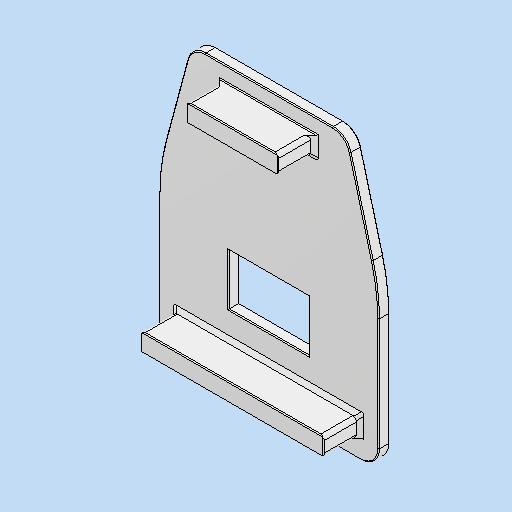
# Autodesk Inventor part: tc-back-panel
Saved by Autodesk Inventor 2025 (Build 290162000, 162)
## iProperties
Created: 2025-06-05
Part Number: tc-back-panel
Material: ABS Plastic
Document SubType Name: Modeling
Designer: queezz
Density: 1.06 g/cm^3
Appearance: Smooth - White
Author: queezz
Autodesk Inventor part; units mm, degrees
ref_plane "YZ Plane" through (0, 0, 0) normal (1, 0, 0) x (0, 1, 0)
ref_plane "XZ Plane" through (0, 0, 0) normal (0, 1, 0) x (-1, 0, 0)
ref_plane "XY Plane" through (0, 0, 0) normal (0, 0, 1) x (1, 0, 0)
sketch "Sketch1" plane through (0, 0, 0) normal (0, 0, 1) x (1, 0, 0)
  line L0 (-60, 75) -> (60, 75)
  line L1 (60, 75) -> (60, -75)
  line L2 (60, -75) -> (-60, -75)
  line L3 (-60, -75) -> (-60, 75)
  point P0 (0, 0)
  point P1 (60, 0)
  point P2 (0, 75)
  dimension "d0" = 120
  dimension "d1" = 150
  constraints: 8 end point, 2 midpoint, 2 parallel, 1 horizontal, 1 horizontal alignment, 1 perpendicular, 1 vertical alignment
  measures "d0" distance of L0.start L0.end
  measures "d1" distance of L0.end L1.end
extrude "Extrusion1" add sketch "Sketch1" along normal blind 6
sketch "Sketch2" plane through (0, 0, 6) normal (0, 0, 1) x (1, 0, 0)
  line L0 (-22, -11.7654) -> (22, -11.7654)
  line L1 (22, -11.7654) -> (22, -39.7654)
  line L2 (22, -39.7654) -> (-22, -39.7654)
  line L3 (-22, -39.7654) -> (-22, -11.7654)
  point P0 (0, 0)
  point P1 (0, -11.7654)
  dimension "d4" = 44
  dimension "d5" = 28
  constraints: 8 end point, 2 parallel, 1 horizontal, 1 midpoint, 1 perpendicular, 1 vertical alignment
  measures "d4" distance of L0.start L0.end
  measures "d5" distance of L0.end L1.end
extrude "PowerPlug" cut sketch "Sketch2" against normal through all
sketch "Sketch3" plane through (0, 0, 6) normal (0, 0, 1) x (1, 0, 0)
  line L0 (22, -11.7654) -> (22, -39.7654) projected
  line L1 (22, -39.7654) -> (-22, -39.7654) projected
  line L2 (-22, -39.7654) -> (-22, -11.7654) projected
  line L3 (-22, -11.7654) -> (22, -11.7654) projected
  line L4 (-60, -75) -> (60, -75) projected
  line L5 (60, -75) -> (60, 75) projected
  line L6 (60, 75) -> (-60, 75) projected
  line L7 (-60, 75) -> (-60, -75) projected
  line L8 (-60, 9.6891) -> (-42.5, 75)
  line L9 (42.5, 75) -> (60, 9.6891)
  line L10 (-42.5, 75) -> (42.5, 75)
  line L11 (60, 75) -> (-60, 75) construction
  point P0 (0, 0)
  point P1 (0, 75)
  dimension "d9" = 15
  dimension "d10" = 85
  constraints: 6 end point, 4 point on line, 1 collinear, 1 equal length, 1 horizontal alignment, 1 midpoint, 1 vertical alignment
  measures "d9" angle of L5 L9
  measures "d10" distance of L9.start L8.end
extrude "Extrusion3" cut sketch "Sketch3" against normal through all contours L7 L6 L8 | L9 L6 L5
fillet "Fillet1" radius 10 4 edges at (60, -75, 3) (-60, -75, 3) (-42.5, 75, 3) (42.5, 75, 3)
fillet "Fillet2" radius 100 2 edges at (60, 9.6891, 3) (-60, 9.6891, 3)
sketch "Sketch5" plane through (0, 0, 6) normal (0, 0, 1) x (1, 0, 0)
  line L0 (-50, -54) -> (50, -54)
  line L1 (50, -54) -> (50, -64)
  line L2 (50, -64) -> (-50, -64)
  line L3 (-50, -64) -> (-50, -54)
  line L4 (-50, -75) -> (50, -75) projected
  line L5 (-25, 67) -> (25, 67)
  line L6 (25, 67) -> (25, 57)
  line L7 (25, 57) -> (-25, 57)
  line L8 (-25, 57) -> (-25, 67)
  line L9 (34.8267, 75) -> (-34.8267, 75) projected
  point P0 (0, 0)
  point P1 (0, -64)
  point P2 (0, 57)
  dimension "d20" = 11
  dimension "d21" = 100
  dimension "d22" = 10
  dimension "d36" = 10
  dimension "d37" = 8
  dimension "d38" = 50
  constraints: 16 end point, 4 parallel, 2 horizontal, 2 midpoint, 2 perpendicular, 2 vertical alignment
  measures "d20" distance between parallel lines of L4 L2
  measures "d21" distance of L1.end L2.end
  measures "d22" distance of L0.end L1.end
  measures "d36" distance of L5.end L6.end
  measures "d37" distance between parallel lines of L9 L5
  measures "d38" distance of L5.start L5.end
extrude "Extrusion4" add sketch "Sketch5" along normal blind 20
chamfer "Chamfer1" distance 0.5 angle 45 24 edges at (0, 75, 6) (-40.9143, 72.9335, 6) (-50.5393, 44.997, 6) (-59.1445, 9.5765, 6) (-60, -34.2381, 6) (-57.0711, -72.0711, 6) (0, -75, 6) (57.0711, -72.0711, 6) (60, -34.2381, 6) (59.1445, 9.5765, 6) (50.5393, 44.997, 6) (40.9143, 72.9335, 6) (0, 75, 0) (-40.9143, 72.9335, 0) (-50.5393, 44.997, 0) (-59.1445, 9.5765, 0) (-60, -34.2381, 0) (-57.0711, -72.0711, 0) (0, -75, 0) (57.0711, -72.0711, 0) (60, -34.2381, 0) (59.1445, 9.5765, 0) (50.5393, 44.997, 0) (40.9143, 72.9335, 0)
chamfer "Chamfer2" distance 0.5 angle 45 8 edges at (0, -11.7654, 6) (-22, -25.7654, 6) (0, -39.7654, 6) (22, -25.7654, 6) (-22, -25.7654, 0) (0, -39.7654, 0) (0, -11.7654, 0) (22, -25.7654, 0)
chamfer "Chamfer3" distance 2 angle 45 6 edges at (0, -54, 6) (-50, -59, 6) (50, -59, 6) (25, 62, 6) (0, 57, 6) (-25, 62, 6)
chamfer "Chamfer4" distance 0.5 angle 45 2 edges at (0, -64, 6) (0, 67, 6)
chamfer "Chamfer5" distance 0.5 angle 45 8 edges at (0, -54, 26) (50, -59, 26) (0, -64, 26) (-50, -59, 26) (0, 67, 26) (-25, 62, 26) (0, 57, 26) (25, 62, 26)
fillet "Fillet3" radius 2 12 edges at (-25, 67, 16.75) (-25, 57, 16.75) (25, 57, 16.75) (25, 67, 16.75) (26, 56, 7) (-26, 56, 7) (50, -54, 16.75) (-50, -54, 16.75) (50, -64, 16.75) (-50, -64, 16.75) (-51, -53, 7) (51, -53, 7)
equation "\"d0\" = width"
equation "\"d1\" = hight"
equation "\"width\" = 120"
equation "\"hight\" = 150"
body "Solid1"
